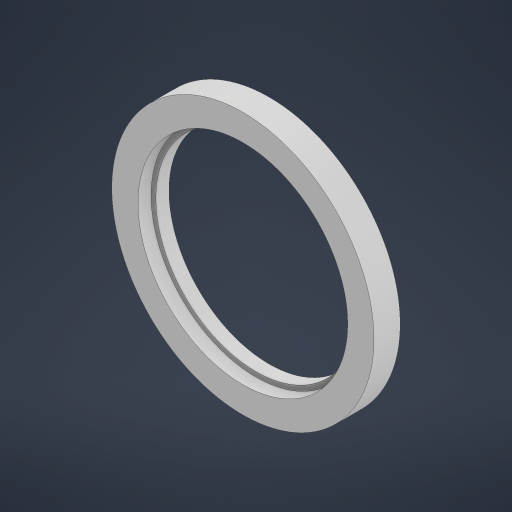
# Autodesk Inventor part: FemaleFlange
Saved by Autodesk Inventor 2023 (Build 270158000, 158)
## iProperties
Created: 2022-10-11
Part Number: FemaleFlange
Material: Generic
Document SubType Name: Modeling
Designer: jdbuo
Density: 1 g/cm^3
Appearance: Default
Author: jdbuo
## iProperties of the stored document FemaleFlange_3DPrint.ipt
Created: 2022-11-10
Part Number: FemaleFlange_3DPrint
Material: Generic
Document SubType Name: Modeling
Designer: jdbuo
Density: 1 g/cm^3
Appearance: Default
Author: jdbuo
Autodesk Inventor part; units mm, degrees
ref_plane "YZ Plane" through (0, 0, 0) normal (1, 0, 0) x (0, 1, 0)
ref_plane "XZ Plane" through (0, 0, 0) normal (0, 1, 0) x (-1, 0, 0)
ref_plane "XY Plane" through (0, 0, 0) normal (0, 0, 1) x (1, 0, 0)
sketch "Sketch1" plane through (0, 0, 0) normal (0, 0, 1) x (1, 0, 0)
  circle A0 centre (0, 0) radius 24.257
  circle A1 centre (0, 0) radius 31.75
  dimension "d0" = 48.514
  dimension "d1" = 63.5
  constraints: 2 centre point, 2 coincident
  measures "d0" diameter of A0
  measures "d1" diameter of A1
extrude "Extrusion1" add sketch "Sketch1" along normal blind 6.35
sketch "Sketch2" plane through (0, 0, 6.35) normal (0, 0, 1) x (1, 0, 0)
  circle A0 centre (0, 0) radius 24.257 projected
  circle A1 centre (0, 0) radius 25.4
  dimension "d4" = 50.8
  constraints: 1 centre point, 1 coincident
  measures "d4" diameter of A1
extrude "Extrusion2" cut sketch "Sketch2" against normal blind 3.175 contours A0 | A1
body "Solid1"
